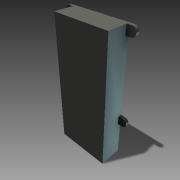
# Autodesk Inventor part: Lisa-M
Saved by Autodesk Inventor 2012 (Build 160160000, 160)
## iProperties
Created: 2013-03-10
Part Number: Lisa-M
Material: Default
Document SubType Name: Modeling
Designer: fixer
Density: 0.748807 g/cm^3
Mass: 11.7 g
Surface Area: 49.5428 cm^2
Volume: 15.6248 cm^3
Author: fixer
Autodesk Inventor part; units mm, degrees
ref_plane "YZ Plane" through (0, 0, 0) normal (1, 0, 0) x (0, 1, 0)
ref_plane "XZ Plane" through (0, 0, 0) normal (0, 1, 0) x (-1, 0, 0)
ref_plane "XY Plane" through (0, 0, 0) normal (0, 0, 1) x (1, 0, 0)
sketch "Sketch1" plane through (0, 0, 0) normal (0, 0, 1) x (1, 0, 0)
  line L0 (12.7, 30.099) -> (-12.7, 30.099)
  line L1 (-12.7, 30.099) -> (-12.7, -30.099)
  line L2 (-12.7, -30.099) -> (12.7, -30.099)
  line L3 (12.7, -30.099) -> (12.7, 30.099)
  point P0 (0, 0)
  point P1 (0, 30.099)
  point P2 (-12.7, 0)
  dimension "d0" = 60.198
  dimension "d1" = 25.4
  constraints: 8 end point, 2 midpoint, 2 parallel, 1 horizontal, 1 horizontal alignment, 1 perpendicular, 1 vertical alignment
  measures "d0" distance of L0.end L1.end
  measures "d1" distance of L0.start L0.end
extrude "Extrusion1" add sketch "Sketch1" along normal blind 10.16
sketch "Sketch2" plane through (0, 0, 0) normal (0, 0, -1) x (-1, 0, 0)
  line L0 (-12.7, 30.099) -> (12.7, 30.099) projected
  line L1 (-12.7, -30.099) -> (-12.7, 30.099) projected
  line L2 (12.7, -30.099) -> (-12.7, -30.099) projected
  arc A0 (-14.732, 30.099) -> (-14.732, 26.035) centre (-14.732, 28.067) ccw
  line L3 (-14.732, 30.099) -> (-12.7, 30.099)
  line L4 (-14.732, 26.035) -> (-12.7, 26.035)
  line L5 (0, 30.099) -> (0, -30.099)
  arc A1 (-14.732, -8.509) -> (-14.732, -12.573) centre (-14.732, -10.541) ccw
  line L6 (-14.732, -8.509) -> (-12.7, -8.509)
  line L7 (-14.732, -12.573) -> (-12.7, -12.573)
  line L8 (-12.7, 30.099) -> (-12.7, 26.035)
  line L9 (-12.7, -8.509) -> (-12.7, -12.573)
  arc A2 (14.732, 26.035) -> (14.732, 30.099) centre (14.732, 28.067) ccw
  line L10 (14.732, 30.099) -> (12.7, 30.099)
  line L11 (14.732, 26.035) -> (12.7, 26.035)
  arc A3 (14.732, -12.573) -> (14.732, -8.509) centre (14.732, -10.541) ccw
  line L12 (14.732, -8.509) -> (12.7, -8.509)
  line L13 (14.732, -12.573) -> (12.7, -12.573)
  line L14 (12.7, 30.099) -> (12.7, 26.035)
  line L15 (12.7, -8.509) -> (12.7, -12.573)
  point P0 (0, 0)
  dimension "d4" = 2.032
  dimension "d5" = 2.032
  dimension "d6" = 42.672
  constraints: 26 end point, 9 symmetric about line, 8 point on circle, 6 tangent, 4 centre point, 2 collinear, 2 midpoint, 2 perpendicular, 1 point on line, 2 other
  measures "d4" radius of A0
  measures "d5" radius of A1
  measures "d6" distance between parallel lines of L7 L3
extrude "Extrusion2" add sketch "Sketch2" against normal blind 1.524 contours L1 L4 A0 L3 | L1 L7 A1 L6 | L11 L14 L10 A2 | L13 L15 L12 A3
body "Solid1"
